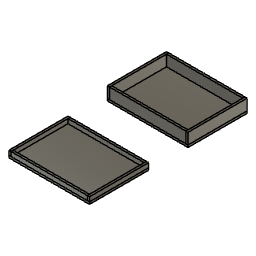
skjalataska v9 (Autodesk Fusion 360 design; units mm, degrees)
Autodesk Fusion 360 part; units mm, degrees
sketch "Sketch1" plane through (0, 0, 0) normal (0, 0, 1) x (1, 0, 0) in component "Toppur"
  line L0 (0, 0) -> (450, 0)
  line L1 (450, 0) -> (450, 330)
  line L2 (450, 330) -> (0, 330)
  line L3 (0, 330) -> (0, 0)
  dimension "d1" = 450
  dimension "d2" = 330
  constraint horizontal L0
  constraint vertical L1
  constraint horizontal L2
  constraint vertical L3
  constraint coincident L0.start L3.end
  measures "d1" distance of L0.start L0.end
  measures "d2" distance of L0 L2
extrude "Extrude1" add sketch "Sketch1" along normal blind 12 makes body 1 in component "Toppur"
sketch "Sketch2" plane through (0, 0, 0) normal (0, 0, -1) x (1, 0, 0) in component "langhlid1"
  line L0 (0, 0) -> (0, -330)
  line L1 (0, -330) -> (450, -330)
  line L2 (450, -330) -> (450, 0)
  line L3 (450, 0) -> (0, 0)
  line L4 (0, -330) -> (12, -330)
  line L5 (12, -330) -> (12, 0)
  line L6 (12, 0) -> (0, 0)
  line L7 (0, 0) -> (0, -330)
  line L8 (450, -330) -> (438, -330)
  line L9 (438, -330) -> (438, 0)
  line L10 (438, 0) -> (450, 0)
  line L11 (450, 0) -> (450, -330)
  dimension "d42" = 12
  dimension "d43" = 12
  constraint horizontal L4
  constraint vertical L5
  constraint horizontal L6
  constraint vertical L7
  constraint coincident L3 L5.end
  constraint coincident L0.end L1.start
  constraint horizontal L8
  constraint vertical L9
  constraint horizontal L10
  constraint vertical L11
  constraint coincident L3 L9.end
  constraint coincident L1.end L2.start
  measures "d42" distance of L5 L7
  measures "d43" distance of L9 L11
extrude "Extrude1'" add sketch "Sketch2" against normal blind 73.3333 separate body contours L1 L2 L3 L8 L9 L10 L11 makes body 2 in component "langhlid1"
sketch "Sketch1 (2)" plane through (0, 0, 0) normal (0, 0, -1) x (1, 0, 0) in component "langhlid2"
  line L0 (0, -330) -> (12, -330)
  line L1 (12, -330) -> (12, 0)
  line L2 (12, 0) -> (0, 0)
  line L3 (0, 0) -> (0, -330)
  line L4 (0, -330) -> (450, -330)
  line L5 (450, 0) -> (450, -330)
  dimension "d53" = 330
  dimension "d54" = 450
  dimension "d55" = 12
  constraint horizontal L0
  constraint vertical L1
  constraint horizontal L2
  constraint vertical L3
  measures "d53" distance of L2 L4
  measures "d54" distance of L3 L5
  measures "d55" distance of L1 L3
extrude "Extrude1''" add sketch "Sketch2" against normal blind 73.3333 separate body contours L0 L1 L3 L4 L5 L6 L7 makes body 3 in component "langhlid2"
combine "Combine1" operation cut target body 3 tool bodies 1 keep tools in component "langhlid2"
combine "Combine2" operation cut target body 2 tool bodies 1 keep tools in component "langhlid1"
sketch "Sketch1 (3)" plane through (0, 0, 0) normal (0, 0, -1) x (1, 0, 0) in component "Skammhlid1"
  line L0 (0, 0) -> (0, -330)
  line L1 (0, -330) -> (450, -330)
  line L2 (450, -330) -> (450, 0)
  line L3 (450, 0) -> (0, 0)
  line L4 (0, 0) -> (450, 0)
  line L5 (450, 0) -> (450, -12)
  line L6 (450, -12) -> (0, -12)
  line L7 (0, -12) -> (0, 0)
  line L8 (0, -330) -> (450, -330)
  line L9 (450, -330) -> (450, -318)
  line L10 (450, -318) -> (0, -318)
  line L11 (0, -318) -> (0, -330)
  dimension "d28" = 12
  dimension "d44" = 12
  constraint horizontal L4
  constraint vertical L5
  constraint horizontal L6
  constraint vertical L7
  constraint coincident L2 L5.end
  constraint coincident L0.start L3.end
  constraint horizontal L8
  constraint vertical L9
  constraint horizontal L10
  constraint vertical L11
  constraint coincident L2 L9.end
  constraint coincident L0.end L1.start
  measures "d28" distance of L4 L6
  measures "d44" distance of L8 L10
extrude "Extrude2" add sketch "Sketch1 (3)" against normal blind 73.3333 separate body contours L0 L2 L3 L4 L5 L6 L7 makes body 4 in component "Skammhlid1"
sketch "Sketch1 (4)" plane through (0, 0, 0) normal (0, 0, -1) x (1, 0, 0) in component "Skammhlid2"
  line L0 (0, 0) -> (0, -330)
  line L1 (0, -330) -> (450, -330)
  line L2 (450, -330) -> (450, 0)
  line L3 (450, 0) -> (0, 0)
  line L4 (450, -330) -> (0, -330)
  line L5 (0, -330) -> (0, -318)
  line L6 (0, -318) -> (450, -318)
  line L7 (450, -318) -> (450, -330)
  dimension "d58" = 12
  constraint horizontal L4
  constraint vertical L5
  constraint horizontal L6
  constraint vertical L7
  constraint coincident L0 L5.end
  constraint coincident L1.end L2.start
  measures "d58" distance of L4 L6
extrude "Extrude1'''" add sketch "Sketch1 (4)" against normal blind 73.3333 separate body contours L0 L1 L2 L4 L5 L6 L7 makes body 5 in component "Skammhlid2"
combine "Combine2'" [suppressed] in component "langhlid2"
combine "Combine4" operation cut target body 4 tool bodies 1 3 2 keep tools in component "Skammhlid1"
combine "Combine3" [suppressed] in component "langhlid1"
combine "Combine1'" operation cut target body 5 tool bodies 1 2 3 keep tools in component "Skammhlid2"
sketch "Sketch1 (5)" plane through (0, 0, 0) normal (0, 0, 1) x (1, 0, 0) in component "Toppur (1)"
  line L0 (0, 0) -> (450, 0)
  line L1 (450, 0) -> (450, 330)
  line L2 (450, 330) -> (0, 330)
  line L3 (0, 330) -> (0, 0)
  dimension "d1_1" = 450
  dimension "d2_1" = 330
  constraint horizontal L0
  constraint vertical L1
  constraint horizontal L2
  constraint vertical L3
  constraint coincident L0.start L3.end
  measures "d1_1" distance of L0.start L0.end
  measures "d2_1" distance of L0 L2
extrude "Extrude1''''" add sketch "Sketch1 (5)" along normal blind 12 separate body makes body 6 in component "Toppur (1)"
sketch "Sketch2 (2)" plane through (0, 0, 0) normal (0, 0, -1) x (1, 0, 0) in component "langhlid1 (1)"
  line L0 (0, 0) -> (0, -330)
  line L1 (0, -330) -> (450, -330)
  line L2 (450, -330) -> (450, 0)
  line L3 (450, 0) -> (0, 0)
  line L4 (0, -330) -> (12, -330)
  line L5 (12, -330) -> (12, 0)
  line L6 (12, 0) -> (0, 0)
  line L7 (0, 0) -> (0, -330)
  line L8 (450, -330) -> (438, -330)
  line L9 (438, -330) -> (438, 0)
  line L10 (438, 0) -> (450, 0)
  line L11 (450, 0) -> (450, -330)
  dimension "d42_1" = 12
  dimension "d43_1" = 12
  constraint horizontal L4
  constraint vertical L5
  constraint horizontal L6
  constraint vertical L7
  constraint coincident L3 L5.end
  constraint coincident L0.end L1.start
  constraint horizontal L8
  constraint vertical L9
  constraint horizontal L10
  constraint vertical L11
  constraint coincident L3 L9.end
  constraint coincident L1.end L2.start
  measures "d42_1" distance of L5 L7
  measures "d43_1" distance of L9 L11
extrude "Extrude1'''''" add sketch "Sketch2 (2)" against normal blind 36.6667 separate body contours L1 L2 L3 L8 L9 L10 L11 makes body 7 in component "langhlid1 (1)"
combine "Combine2''" operation cut target body 7 tool bodies 1 keep tools in component "langhlid1 (1)"
combine "Combine3'" [suppressed] in component "langhlid1 (1)"
sketch "Sketch1 (6)" plane through (0, 0, 0) normal (0, 0, -1) x (1, 0, 0) in component "langhlid2 (1)"
  line L0 (0, -330) -> (12, -330)
  line L1 (12, -330) -> (12, 0)
  line L2 (12, 0) -> (0, 0)
  line L3 (0, 0) -> (0, -330)
  line L4 (0, -330) -> (450, -330)
  line L5 (450, 0) -> (450, -330)
  dimension "d53_1" = 330
  dimension "d54_1" = 450
  dimension "d55_1" = 12
  constraint horizontal L0
  constraint vertical L1
  constraint horizontal L2
  constraint vertical L3
  measures "d53_1" distance of L2 L4
  measures "d54_1" distance of L3 L5
  measures "d55_1" distance of L1 L3
extrude "Extrude1''''''" add sketch "Sketch2" against normal blind 36.6667 separate body contours L0 L1 L3 L4 L5 L6 L7 makes body 8 in component "langhlid2 (1)"
combine "Combine1''" operation cut target body 8 tool bodies 1 keep tools in component "langhlid2 (1)"
combine "Combine2'''" [suppressed] in component "langhlid2 (1)"
sketch "Sketch1 (7)" plane through (0, 0, 0) normal (0, 0, -1) x (1, 0, 0) in component "Skammhlid2 (1)"
  line L0 (0, 0) -> (0, -330)
  line L1 (0, -330) -> (450, -330)
  line L2 (450, -330) -> (450, 0)
  line L3 (450, 0) -> (0, 0)
  line L4 (450, -330) -> (0, -330)
  line L5 (0, -330) -> (0, -318)
  line L6 (0, -318) -> (450, -318)
  line L7 (450, -318) -> (450, -330)
  dimension "d58_1" = 12
  constraint horizontal L4
  constraint vertical L5
  constraint horizontal L6
  constraint vertical L7
  constraint coincident L0 L5.end
  constraint coincident L1.end L2.start
  measures "d58_1" distance of L4 L6
extrude "Extrude1'''''''" add sketch "Sketch1 (7)" against normal blind 36.6667 separate body contours L0 L1 L2 L4 L5 L6 L7 makes body 9 in component "Skammhlid2 (1)"
combine "Combine1'''" operation cut target body 9 tool bodies 1 2 3 keep tools in component "Skammhlid2 (1)"
sketch "Sketch1 (8)" plane through (0, 0, 0) normal (0, 0, -1) x (1, 0, 0) in component "Skammhlid1 (1)"
  line L0 (0, 0) -> (0, -330)
  line L1 (0, -330) -> (450, -330)
  line L2 (450, -330) -> (450, 0)
  line L3 (450, 0) -> (0, 0)
  line L4 (0, 0) -> (450, 0)
  line L5 (450, 0) -> (450, -12)
  line L6 (450, -12) -> (0, -12)
  line L7 (0, -12) -> (0, 0)
  line L8 (0, -330) -> (450, -330)
  line L9 (450, -330) -> (450, -318)
  line L10 (450, -318) -> (0, -318)
  line L11 (0, -318) -> (0, -330)
  dimension "d28_1" = 12
  dimension "d44_1" = 12
  constraint horizontal L4
  constraint vertical L5
  constraint horizontal L6
  constraint vertical L7
  constraint coincident L2 L5.end
  constraint coincident L0.start L3.end
  constraint horizontal L8
  constraint vertical L9
  constraint horizontal L10
  constraint vertical L11
  constraint coincident L2 L9.end
  constraint coincident L0.end L1.start
  measures "d28_1" distance of L4 L6
  measures "d44_1" distance of L8 L10
extrude "Extrude2'" add sketch "Sketch1 (8)" against normal blind 36.6667 separate body contours L0 L2 L3 L4 L5 L6 L7 makes body 10 in component "Skammhlid1 (1)"
combine "Combine4'" operation cut target body 10 tool bodies 1 3 2 keep tools in component "Skammhlid1 (1)"
sketch "Sketch4" plane through (0, 0, 12) normal (0, 0, 1) x (-1, 0, 0)
  line L0 (-1100, -330) -> (-1100, 0)
  line L1 (-1100, 0) -> (-1550, 0)
  line L2 (-1550, 0) -> (-1550, -330)
  line L3 (-1550, -330) -> (-1100, -330)
  line L4 (-1550, -330) -> (-1100, -330)
  line L5 (-1550, 0) -> (-1550, -330)
  line L6 (-1100, 0) -> (-1550, 0)
  line L7 (-1100, -330) -> (-1100, 0)
  line L8 (-1063, -330) -> (-1063, 0)
  line L9 (-1063, -330) -> (-1001.6667, -330)
  line L10 (-1063, 0) -> (-1001.6667, 0)
  line L11 (-1001.6667, -330) -> (-1001.6667, 0)
  line L12 (-1612, 0) -> (-1612, -330)
  line L13 (-1612, -330) -> (-1673.3333, -330)
  line L14 (-1673.3333, 0) -> (-1673.3333, -330)
  line L15 (-1612, 0) -> (-1673.3333, 0)
  line L16 (-1112, -362) -> (-1112, -423.3333)
  line L17 (-1538, -362) -> (-1112, -362)
  line L18 (-1538, -423.3333) -> (-1112, -423.3333)
  line L19 (-1538, -423.3333) -> (-1538, -362)
  line L20 (-1538, 37) -> (-1538, 98.3333)
  line L21 (-1112, 98.3333) -> (-1538, 98.3333)
  line L22 (-1112, 98.3333) -> (-1112, 37)
  line L23 (-1112, 37) -> (-1538, 37)
  line L24 (-1112, 188) -> (-1112, 163.3333)
  line L25 (-1538, 188) -> (-1112, 188)
  line L26 (-1538, 163.3333) -> (-1112, 163.3333)
  line L27 (-1538, 163.3333) -> (-1538, 188)
  line L28 (-1587, 550) -> (-1587, 220)
  line L29 (-1587, 220) -> (-1611.6667, 220)
  line L30 (-1611.6667, 550) -> (-1611.6667, 220)
  line L31 (-1587, 550) -> (-1611.6667, 550)
  line L32 (-1063, 220) -> (-1063, 550)
  line L33 (-1063, 220) -> (-1038.3333, 220)
  line L34 (-1063, 550) -> (-1038.3333, 550)
  line L35 (-1038.3333, 220) -> (-1038.3333, 550)
  line L36 (-1538, 577) -> (-1538, 601.6667)
  line L37 (-1112, 601.6667) -> (-1538, 601.6667)
  line L38 (-1112, 601.6667) -> (-1112, 577)
  line L39 (-1112, 577) -> (-1538, 577)
  line L40 (-1550, 220) -> (-1100, 220)
  line L41 (-1550, 550) -> (-1550, 220)
  line L42 (-1100, 550) -> (-1550, 550)
  line L43 (-1100, 220) -> (-1100, 550)
component "Toppur" placed x (1, 0, 0) y (0, 1, 0) z (0, 0, 1) at (0, 0, 0)
component "langhlid1" placed x (1, 0, 0) y (0, 1, 0) z (0, 0, 1) at (0, 0, 0)
component "langhlid2" placed x (1, 0, 0) y (0, 1, 0) z (0, 0, 1) at (0, 0, 0)
component "Skammhlid1" placed x (1, 0, 0) y (0, 1, 0) z (0, 0, 1) at (0, 0, 0)
component "Skammhlid2" placed x (1, 0, 0) y (0, 1, 0) z (0, 0, 1) at (0, 0, 0)
component "DFX Módel" placed x (1, 0, 0) y (0, 1, 0) z (0, 0, 1) at (0, 0, 0)
component "AnHandfangs" placed x (1, 0, 0) y (0, 1, 0) z (0, 0, 1) at (0, 0, 0)
component "DXF AnHandfangs" placed x (1, 0, 0) y (0, 1, 0) z (0, 0, 1) at (0, 0, 0)
component "langhlid2" placed x (0, 0, 1) y (0, 1, 0) z (-1, 0, 0) at (1075, 0, 0) in component "DFX Módel"
component "Skammhlid1" placed x (1, 0, 0) y (0, 0, 1) z (0, -1, 0) at (1100, -25, 0) in component "DFX Módel"
component "Skammhlid2" placed x (1, 0, 0) y (0, 0, -1) z (0, 1, 0) at (1100, 350, 330) in component "DFX Módel"
component "langhlid1" placed x (0, 0, -1) y (0, 1, 0) z (1, 0, 0) at (1600, 0, 450) in component "DFX Módel"
component "Toppur" placed x (1, 0, 0) y (0, 1, 0) z (0, 0, 1) at (1100, 0, 0) in component "DFX Módel"
component "Toppur (1)" placed x (1, 0, 0) y (0, 1, 0) z (0, 0, 1) at (0, -550, 0) in component "AnHandfangs"
component "langhlid1 (1)" placed x (1, 0, 0) y (0, 1, 0) z (0, 0, 1) at (0, -550, 0) in component "AnHandfangs"
component "langhlid2 (1)" placed x (1, 0, 0) y (0, 1, 0) z (0, 0, 1) at (0, -550, 0) in component "AnHandfangs"
component "Skammhlid2 (1)" placed x (1, 0, 0) y (0, 1, 0) z (0, 0, 1) at (0, -550, 0) in component "AnHandfangs"
component "Skammhlid1 (1)" placed x (1, 0, 0) y (0, 1, 0) z (0, 0, 1) at (0, -550, 0) in component "AnHandfangs"
component "Toppur (1)" placed x (1, 0, 0) y (0, 1, 0) z (0, 0, 1) at (1100, -550, 0) in component "DXF AnHandfangs"
component "langhlid1 (1)" placed x (0, 0, -1) y (0, 1, 0) z (1, 0, 0) at (1575, -550, 450) in component "DXF AnHandfangs"
component "langhlid2 (1)" placed x (0, 0, 1) y (0, 1, 0) z (-1, 0, 0) at (1075, -550, 0) in component "DXF AnHandfangs"
component "Skammhlid2 (1)" placed x (1, 0, 0) y (0, 0, -1) z (0, 1, 0) at (1100, -200, 330) in component "DXF AnHandfangs"
component "Skammhlid1 (1)" placed x (1, 0, 0) y (0, 0, 1) z (0, -1, 0) at (1100, -565, 0) in component "DXF AnHandfangs"
equation "d1 = lengd"
equation "d2 = hæð"
equation "lengd = 450 mm"
equation "hæð = 330 mm"
equation "breidd = 110 mm"
equation "þykkt = 12 mm"
equation "d7 = þykkt"
equation "d28 = þykkt"
equation "d42 = þykkt"
equation "d43 = þykkt"
equation "d44 = þykkt"
equation "d45 = -2 * breidd / 3"
equation "d49 = -2 * breidd / 3"
equation "d53 = hæð"
equation "d54 = lengd"
equation "d55 = þykkt"
equation "d56 = -2 * breidd / 3"
equation "d58 = þykkt"
equation "d59 = -2 * breidd / 3"
equation "d1_1 = lengd"
equation "d2_1 = hæð"
equation "d7_1 = þykkt"
equation "d42_1 = þykkt"
equation "d43_1 = þykkt"
equation "d49_1 = -breidd / 3"
equation "d53_1 = hæð"
equation "d54_1 = lengd"
equation "d55_1 = þykkt"
equation "d56_1 = -breidd / 3"
equation "d58_1 = þykkt"
equation "d59_1 = -breidd / 3"
equation "d28_1 = þykkt"
equation "d44_1 = þykkt"
equation "d45_1 = -breidd / 3"
named bodies: "Framhlið", "Hlið2"
